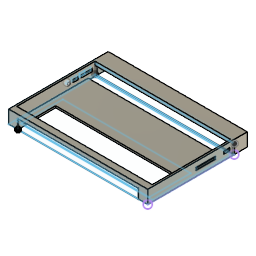
Dół (Autodesk Fusion 360 design; units mm, degrees)
part number: 2025-11-11-11-26-44-034
Autodesk Fusion 360 part; units mm, degrees
note: some values were not read from the file. Set by a fixed rule: which sketch regions a step uses.
sketch "Szkic1" plane through (0, 0, 0) normal (0, 0, 1) x (1, 0, 0)
  line L0 (-25, 50.8) -> (345, 50.8)
  line L1 (345, 50.8) -> (345, -179.1)
  line L2 (345, -179.1) -> (-25, -179.1)
  line L3 (-25, -179.1) -> (-25, 50.8)
  line L4 (-20, 45.8) -> (340, 45.8)
  line L5 (340, 45.8) -> (340, -162.2)
  line L6 (340, -162.2) -> (-20, -162.2)
  line L7 (-20, -162.2) -> (-20, 45.8)
  line L8 (-10, -50) -> (330, -50)
  line L9 (330, -50) -> (330, -160)
  line L10 (330, -160) -> (-10, -160)
  line L11 (-10, -160) -> (-10, -50)
  dimension "d1" = 370
  dimension "d2" = 229.9
  dimension "d3" = 360
  dimension "d4" = 208
  dimension "d5" = 5
  dimension "d6" = 16.9
  constraint horizontal L0
  constraint vertical L1
  constraint horizontal L2
  constraint vertical L3
  constraint horizontal L4
  constraint vertical L5
  constraint horizontal L6
  constraint vertical L7
  constraint horizontal L8
  constraint vertical L9
  constraint horizontal L10
  constraint vertical L11
  measures "d1" distance of L0.start L0.end
  measures "d2" distance of L0.start L2.end
  measures "d3" distance of L4.start L4.end
  measures "d4" distance of L4.start L6.end
  measures "d5" distance of L3 L7
  measures "d6" distance of L2 L6
extrude "Wyciągnięcie proste1" add sketch "Szkic1" along normal blind 35 contours L0 L1 L2 L3
extrude "Wyciągnięcie proste2" add sketch "Szkic1" along normal blind 5 contours L4 L5 L6 L7 | L8 L9 L10 L11
sketch "Szkic2" plane through (-25, 0, 0) normal (-1, 0, 0) x (0, -1, 0)
  line L0 (-50.8, 0) -> (179.1, 0)
  line L1 (179.1, 0) -> (179.1, 35)
  line L2 (179.1, 35) -> (-50.8, 35)
  line L3 (-50.8, 35) -> (-50.8, 0)
  line L4 (-22.9208, 21.9096) -> (-8.9208, 21.9096)
  line L5 (-8.9208, 21.9096) -> (-8.9208, 14.9096)
  line L6 (-8.9208, 14.9096) -> (-22.9208, 14.9096)
  line L7 (-22.9208, 14.9096) -> (-22.9208, 21.9096)
  line L8 (-38.9208, 21.9096) -> (-8.9208, 21.9096)
  line L9 (-8.9208, 21.9096) -> (-8.9208, 14.9096)
  line L10 (-8.9208, 14.9096) -> (-38.9208, 14.9096)
  line L11 (-38.9208, 14.9096) -> (-38.9208, 21.9096)
  line L12 (-1.4208, 21.9096) -> (12.5792, 21.9096)
  line L13 (12.5792, 21.9096) -> (12.5792, 14.9096)
  line L14 (12.5792, 14.9096) -> (-1.4208, 14.9096)
  line L15 (-1.4208, 14.9096) -> (-1.4208, 21.9096)
  circle A0 centre (24.0792, 18.4096) radius 3.25
  dimension "d11" = 14
  dimension "d12" = 7
  dimension "d13" = 30
  dimension "d14" = 7
  dimension "d15" = 14
  dimension "d16" = 7
  dimension "d17" = 7.5
  dimension "d18" = 6.5
  dimension "d19" = 11.5
  constraint horizontal L4
  constraint vertical L5
  constraint horizontal L6
  constraint vertical L7
  constraint horizontal L8
  constraint vertical L9
  constraint horizontal L10
  constraint vertical L11
  constraint horizontal L12
  constraint vertical L13
  constraint horizontal L14
  constraint vertical L15
  measures "d11" distance of L4.start L4.end
  measures "d12" distance of L4.start L6.end
  measures "d13" distance of L4.end L8.start
  measures "d14" distance of L10.end L8.start
  measures "d15" distance of L12.end L12.start
  measures "d16" distance of L14.end L12.start
  measures "d17" distance of L9 L15
  measures "d18" diameter of A0
  measures "d19" distance of L13 A0.centre
extrude "Wyciągnięcie proste3" cut sketch "Szkic2" against normal blind 3 contours L4 L5 L6 L7 L8 L9 L10 | L12 L13 L14 L15 | A0
extrude "Wyciągnięcie proste4" cut 3 faces at (-22, 18.2542, 17.2429) (-22, -3.2458, 19.5763) (-22, -23.249, 17.192) along direction (1, 0, 0) blind 2
sketch "Szkic3" plane through (345, 0, 0) normal (1, 0, 0) x (0, 1, 0)
  line L0 (-179.1, 0) -> (50.8, 0)
  line L1 (50.8, 0) -> (50.8, 35)
  line L2 (50.8, 35) -> (-179.1, 35)
  line L3 (-179.1, 35) -> (-179.1, 0)
  line L4 (-50, 20.91) -> (0, 20.91)
  line L5 (0, 20.91) -> (0, 14.91)
  line L6 (0, 14.91) -> (-50, 14.91)
  line L7 (-50, 14.91) -> (-50, 20.91)
  line L8 (50.8, 0) -> (-179.1, 0)
  dimension "d24" = 50
  dimension "d25" = 6
  dimension "d26" = 14.91
  constraint horizontal L4
  constraint vertical L5
  constraint horizontal L6
  constraint vertical L7
  measures "d24" distance of L4.start L4.end
  measures "d25" distance of L4.start L6.end
  measures "d26" distance of L6 L8
extrude "Wyciągnięcie proste5" cut sketch "Szkic3" against normal blind 50 contours L4 L5 L6 L7
extrude "Wyciągnięcie proste6" cut sketch "Szkic2" against normal blind 450 contours L7 L8 L10 L11
sketch "Szkic4" plane through (0, -179.1, 0) normal (0, -1, 0) x (1, 0, 0)
  line L0 (-25, 0) -> (345, 0)
  line L1 (345, 0) -> (345, 35)
  line L2 (345, 35) -> (-25, 35)
  line L3 (-25, 35) -> (-25, 0)
  line L4 (0, 0) -> (320, 0)
  line L5 (320, 0) -> (320, 24.5591)
  line L6 (320, 24.5591) -> (0, 24.5591)
  line L7 (0, 24.5591) -> (0, 0)
  dimension "d31" = 320
  dimension "d32" = 25
  constraint horizontal L4
  constraint vertical L5
  constraint horizontal L6
  constraint vertical L7
  constraint coincident L0 L4.start
  measures "d31" distance of L5.end L6.end
  measures "d32" distance of L1 L5
extrude "Wyciągnięcie proste7" cut sketch "Szkic4" against normal blind 100 contours L0 L4 L5 L6 L7
extrude "Wyciągnięcie proste8" cut sketch "Szkic4" against normal blind 120 contours L0 L4 L5 L6 L7
extrude "Wyciągnięcie proste9" add sketch "Szkic1" along normal blind 5 contours L8 L9 L10 L11
extrude "Wyciągnięcie proste10" cut sketch "Szkic4" against normal blind 100 contours L0 L4 L5 L6 L7
sketch "Szkic5" plane through (0, 50.8, 0) normal (0, 1, 0) x (-1, 0, 0)
  line L0 (-345, 0) -> (25, 0)
  line L1 (25, 0) -> (25, 35)
  line L2 (25, 35) -> (-345, 35)
  line L3 (-345, 35) -> (-345, 0)
  line L4 (-345, 25.3824) -> (25, 25.3824)
  line L5 (25, 25.3824) -> (25, 0)
  line L6 (25, 0) -> (-345, 0)
  line L7 (-345, 0) -> (-345, 25.3824)
  line L8 (-340, 25.3824) -> (20, 25.3824)
  line L9 (20, 25.3824) -> (20, 0)
  line L10 (20, 0) -> (-340, 0)
  line L11 (-340, 0) -> (-340, 25.3824)
  dimension "d41" = 360
  dimension "d42" = 5
  constraint horizontal L4
  constraint vertical L5
  constraint horizontal L6
  constraint vertical L7
  constraint coincident L0.end L1.start
  constraint coincident L3 L4.start
  constraint horizontal L8
  constraint vertical L9
  constraint horizontal L10
  constraint vertical L11
  constraint coincident L6 L9.end
  constraint coincident L4 L8.start
  measures "d41" distance of L8.start L8.end
  measures "d42" distance of L5 L9
extrude "Wyciągnięcie proste11" add sketch "Szkic5" along normal blind 15 contours L0 L4 L6 L8 L9 L10 L11
extrude "Wyciągnięcie proste12" cut 1 faces at (220, 65.8, 16.9216) along direction (0, -1, 0) blind 18
extrude "Wyciągnięcie proste13" cut 1 faces at (220, 47.8, 16.9216) along direction (0, -1, 0) blind 20
extrude "Wyciągnięcie proste14" add sketch "Szkic5" along normal blind 35 contours L0 L3 L4 L6 L7 L11 | L1 L2 L3 L4 L8 | L0 L1 L4 L5 L6 L9
equation "d22 = 0 mm - 2.00 mm"
